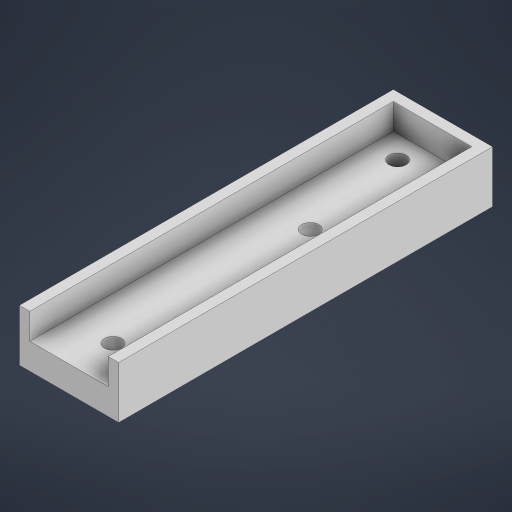
# Autodesk Inventor part: wing hole drill
Saved by Autodesk Inventor 2024 (Build 280153000, 153)
## iProperties
Created: 2024-02-08
Part Number: wing hole drill
Material: Generic
Document SubType Name: Modeling
Designer: elite
Density: 1 g/cm^3
Appearance: Default
Author: elite
Autodesk Inventor part; units mm, degrees
ref_plane "YZ Plane" through (0, 0, 0) normal (1, 0, 0) x (0, 1, 0)
ref_plane "XZ Plane" through (0, 0, 0) normal (0, 1, 0) x (-1, 0, 0)
ref_plane "XY Plane" through (0, 0, 0) normal (0, 0, 1) x (1, 0, 0)
sketch "Sketch1" plane through (0, 0, 0) normal (0, 1, 0) x (-1, 0, 0)
  line L0 (0, 0) -> (19.177, 0)
  line L1 (19.177, 0) -> (19.177, -88.9)
  line L2 (19.177, -88.9) -> (0, -88.9)
  line L3 (0, -88.9) -> (0, 0)
  line L4 (0, -88.9) -> (0, -91.44)
  line L5 (0, -91.44) -> (19.177, -91.44)
  line L6 (19.177, -91.44) -> (19.177, -88.9)
  line L7 (19.177, 0) -> (21.717, 0)
  line L8 (21.717, 0) -> (21.717, -91.44)
  line L9 (21.717, -91.44) -> (19.177, -91.44)
  line L10 (0, -91.44) -> (-2.54, -91.44)
  line L11 (-2.54, -91.44) -> (-2.54, 0)
  line L12 (-2.54, 0) -> (0, 0)
  dimension "d0" = 19.177
  dimension "d1" = 88.9
  dimension "d2" = 2.54
  dimension "d8" = 2.54
  dimension "d9" = 2.54
  constraints: 26 end point, 6 perpendicular, 3 horizontal, 3 parallel, 1 vertical
  measures "d0" distance of L1.end L2.end
  measures "d1" distance of L0.end L1.end
  measures "d2" distance of L2.end L4.end
  measures "d8" distance of L0.end L7.end
  measures "d9" distance of L4.end L10.end
extrude "Extrusion1" add sketch "Sketch1" along normal blind 6.35
sketch "Sketch4" plane through (0, 6.35, 0) normal (0, 1, 0) x (1, 0, 0)
  line L0 (-21.717, 0) -> (2.54, 0) projected
  line L1 (-21.717, 0) -> (-19.177, 0)
  line L2 (2.54, 91.44) -> (-21.717, 91.44) projected
  line L3 (-21.717, 0) -> (-21.717, 91.44)
  line L4 (-21.717, 91.44) -> (2.54, 91.44)
  line L5 (2.54, 91.44) -> (2.54, 0)
  line L6 (0, 0) -> (0, 88.9)
  line L7 (0, 88.9) -> (-19.177, 88.9)
  line L8 (-19.177, 88.9) -> (-19.177, 0)
  line L9 (-19.177, 0) -> (-21.717, 0)
  dimension "d12" = 2.54
  dimension "d13" = 88.9
  constraints: 16 end point, 3 perpendicular, 2 collinear, 1 horizontal, 1 point on line, 1 vertical
  measures "d12" distance of L0.start L1.end
  measures "d13" distance of L6.start L6.end
extrude "Extrusion3" add sketch "Sketch4" along normal blind 6.35 contours L3 L2 L5 L0 L6 L7 L8
sketch "Sketch5" plane through (0, 6.35, 0) normal (0, 1, 0) x (1, 0, 0)
  line L0 (-19.177, 88.9) -> (0, 88.9) projected
  line L1 (-19.177, 88.9) -> (-12.6238, 88.9)
  line L2 (-12.6238, 88.9) -> (-12.6238, 83.3882)
  circle A0 centre (-12.6238, 83.3882) radius 2.1082
  line L3 (-12.6238, 83.3882) -> (-8.5852, 83.3882)
  line L4 (-8.5852, 83.3882) -> (-8.5852, 57.9882)
  circle A1 centre (-8.5852, 57.9882) radius 2.1082
  line L5 (-8.5852, 57.9882) -> (-8.5852, 9.7282)
  circle A2 centre (-8.5852, 9.7282) radius 2.1082
  point P0 (0, 0)
  dimension "d16" = 6.5532
  dimension "d17" = 5.5118
  dimension "d18" = 4.2164
  dimension "d19" = 4.0386
  dimension "d20" = 25.4
  dimension "d21" = 4.2164
  dimension "d22" = 48.26
  dimension "d23" = 4.2164
  constraints: 10 end point, 3 centre point, 3 coincident, 2 perpendicular, 1 horizontal, 1 point on line, 1 vertical
  measures "d16" distance of L0.start L1.end
  measures "d17" distance of L1.end L2.end
  measures "d18" diameter of A0
  measures "d19" distance of L3.start L3.end
  measures "d20" distance of L3.end L4.end
  measures "d21" diameter of A1
  measures "d22" distance of L5.start L5.end
  measures "d23" diameter of A2
extrude "Extrusion4" cut sketch "Sketch5" against normal blind 6.35
body "Solid1"
